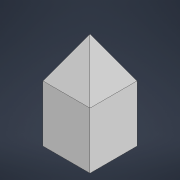
# Autodesk Inventor part: 110033226_ipt_06_小尖頂
Saved by Autodesk Inventor 2022 (Build 260153000, 153)
## iProperties
Created: 2022-06-22
Part Number: 110033226_ipt_06_小尖頂
Material: 一般
Document SubType Name: Modeling
Designer: User
Density: 1 g/cm^3
Appearance: 預設
Author: User
Autodesk Inventor part; units mm, degrees
ref_plane "YZ Plane" through (0, 0, 0) normal (1, 0, 0) x (0, 1, 0)
ref_plane "XZ Plane" through (0, 0, 0) normal (0, 1, 0) x (-1, 0, 0)
ref_plane "XY Plane" through (0, 0, 0) normal (0, 0, 1) x (1, 0, 0)
sketch "草圖1" plane through (0, 0, 0) normal (0, 1, 0) x (-1, 0, 0)
  line L0 (5, 5) -> (-5, 5)
  line L1 (-5, 5) -> (-5, -5)
  line L2 (-5, -5) -> (5, -5)
  line L3 (5, -5) -> (5, 5)
  circle A0 centre (2.5, 2.5) radius 1.7
  circle A1 centre (-2.5, 2.5) radius 1.7
  circle A2 centre (2.5, -2.5) radius 1.7
  circle A3 centre (-2.5, -2.5) radius 1.7
  point P0 (0, 0)
  point P1 (0, -5)
  point P2 (5, 0)
  dimension "d0" = 10
  dimension "d1" = 10
  dimension "d2" = 3.4
  dimension "d3" = 2.5
  dimension "d4" = 2.5
  dimension "d7" = 5
  dimension "d10" = 5
  constraints: 8 end point, 4 centre point, 2 horizontal, 2 midpoint, 2 parallel, 1 horizontal alignment, 1 perpendicular, 1 vertical, 1 vertical alignment, 6 other
  measures "d0" distance of L2.end L1.end
  measures "d1" distance of L0.end L1.end
  measures "d2" diameter of A0
  measures "d3" distance from line of L3 A0.centre
  measures "d4" distance from line of L0 A0.centre
  measures "d7" distance of A0.centre A1.centre
  measures "d10" distance of A0.centre A2.centre
extrude "擠出1" add sketch "草圖1" along normal blind 12 contours L3 L2 L1 L0 | A0 | A1 | A2 | A3
sketch "草圖2" plane through (0, 12, 0) normal (0, 1, 0) x (1, 0, 0)
  line L0 (5, -5) -> (5, 5) projected
  line L1 (5, 5) -> (-5, 5) projected
  line L2 (-5, 5) -> (-5, -5) projected
  line L3 (-5, -5) -> (5, -5) projected
  point P0 (0, 0)
extrude "擠出2" add sketch "草圖2" along normal blind 12 draft -30
